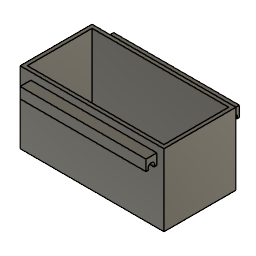
boite_v0.1 (Autodesk Fusion 360 design; units mm, degrees)
Autodesk Fusion 360 part; units mm, degrees
note: some values were not read from the file. Set by a fixed rule: which sketch regions a step uses.
sketch "Esquisse1" plane through (0, 0, 0) normal (0, 0, 1) x (1, 0, 0)
  line L0 (-20, 20) -> (180, 20)
  line L1 (180, 20) -> (180, -80)
  line L2 (180, -80) -> (-20, -80)
  line L3 (-20, -80) -> (-20, 20)
  dimension "d7" = 200
  dimension "d8" = 100
  constraint horizontal L0
  constraint vertical L1
  constraint horizontal L2
  constraint vertical L3
  measures "d7" distance of L0.start L0.end
  measures "d8" distance of L0.start L2.end
sketch "Esquisse2" plane through (180, 0, 0) normal (1, 0, 0) x (0, 1, 0)
  line L0 (-80, 0) -> (20, 0)
  line L1 (20, 0) -> (20, 100)
  line L2 (20, 100) -> (-80, 100)
  line L3 (-80, 100) -> (-80, 0)
  circle A0 centre (-105, 61.7948) radius 25
  dimension "d13" = 50
  constraint tangent L3 A0
  measures "d13" diameter of A0
sketch "Esquisse3" plane through (0, 0, 0) normal (0, 0, 1) x (1, 0, 0)
  line L0 (100, 50) -> (-100, 50)
  line L1 (-100, 50) -> (-100, -50)
  line L2 (-100, -50) -> (100, -50)
  line L3 (100, -50) -> (100, 50)
  line L4 (100, 50) -> (-100, -50) construction
  line L5 (-100, 50) -> (100, -50) construction
  dimension "d16" = 200
  dimension "d17" = 100
  constraint horizontal L0
  constraint perpendicular L0 L1
  constraint parallel L0 L2
  constraint parallel L1 L3
  constraint coincident L4 origin
  constraint coincident L5 origin
  measures "d16" distance of L1.end L2.end
  measures "d17" distance of L0.end L1.end
extrude "Extrusion3" add sketch "Esquisse3" along normal blind 100
shell "Coque2" thickness 5 removed faces 1 at (-33.3333, 16.6667, 100)
sketch "Esquisse4" plane through (0, -50, 0) normal (0, -1, 0) x (1, 0, 0)
  line L0 (-100, 0) -> (100, 0)
  line L1 (100, 0) -> (100, 100)
  line L2 (100, 100) -> (-100, 100)
  line L3 (-100, 100) -> (-100, 0)
  line L4 (-85, 90) -> (90, 90)
  line L5 (90, 90) -> (90, 75)
  line L6 (90, 75) -> (-85, 75)
  line L7 (-85, 90) -> (-85, 75)
  constraint perpendicular L4 L5
  constraint perpendicular L5 L6
  constraint perpendicular L6 L7
extrude "Extrusion4" add sketch "Esquisse4" along normal blind 15 contours L4 L5 L6 L7
sketch "Esquisse5" plane through (90, 0, 0) normal (1, 0, 0) x (0, 1, 0)
  line L0 (-50, 75) -> (-50, 90)
  line L1 (-50, 90) -> (-65, 90)
  line L2 (-65, 90) -> (-65, 75)
  line L3 (-65, 75) -> (-50, 75)
  circle A0 centre (-57.5, 77.5132) radius 4.5
  dimension "d23" = 9
  measures "d23" diameter of A0
extrude "Extrusion5" cut sketch "Esquisse5" against normal blind 180 contours L3 A0 picked at (-57.7191, 77.5283)
mirror "Symétrie miroir1" about plane through (0, 0, 0) normal (0, 1, 0) of "Extrusion4", "Extrusion5"
extrude "Extrusion2" [suppressed]
equation "largeur = 100 mm"
equation "hauteur = 100 mm"
equation "longueur = 200 mm"
equation "epaisseurb = 5 mm"
equation "rayon = 50 mm"
equation "fixation = 5 mm"
equation "d7 = longueur"
equation "d8 = largeur"
equation "epaisseurinterieur = 5 mm"
equation "d13 = rayon"
equation "d14 = -longueur"
equation "d16 = longueur"
equation "d17 = largeur"
equation "d18 = hauteur"
equation "d20 = epaisseurinterieur"
